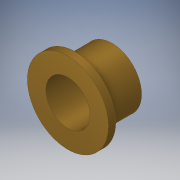
# Autodesk Inventor part: 3_8_FLANGED_BUSHING
Saved by Autodesk Inventor 2019.4 (Build 234330000, 330)
## iProperties
Created: 2020-01-27
Part Number: 3_8_FLANGED_BUSHING
Material: Brass, Soft Yellow
Document SubType Name: Modeling
Designer: mavericks
Density: 8.47 g/cm^3
Appearance: Brass - Satin
Author: mavericks
Autodesk Inventor part; units mm, degrees
ref_plane "YZ Plane" through (0, 0, 0) normal (1, 0, 0) x (0, 1, 0)
ref_plane "XZ Plane" through (0, 0, 0) normal (0, 1, 0) x (-1, 0, 0)
ref_plane "XY Plane" through (0, 0, 0) normal (0, 0, 1) x (1, 0, 0)
sketch "Sketch1" plane through (0, 0, 0) normal (0, 0, 1) x (1, 0, 0)
  circle A0 centre (0, 0) radius 6.3627
  circle A1 centre (0, 0) radius 4.7625
  dimension "d0" = 12.7254
  dimension "d1" = 9.525
  constraints: 3 coincident, 2 centre point
  measures "d0" diameter of A0
  measures "d1" diameter of A1
extrude "Extrusion1" add sketch "Sketch1" along normal blind 9.525
sketch "Sketch2" plane through (0, 0, 9.525) normal (0, 0, 1) x (1, 0, 0)
  circle A0 centre (0, 0) radius 8.7376
  circle A1 centre (0, 0) radius 4.7625 projected
  circle A2 centre (0, 0) radius 6.3627 projected
  dimension "d4" = 17.4752
  constraints: 1 centre point, 1 coincident
  measures "d4" diameter of A0
extrude "Extrusion2" add sketch "Sketch2" against normal blind 1.5875 contours A0
body "Solid1"
